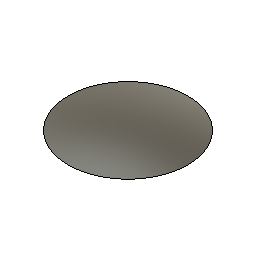
form (Autodesk Fusion 360 design; units mm, degrees)
Autodesk Fusion 360 part; units mm, degrees
sphere "Prymityw sfery1" add diameter 1500 placed x (1, 0, 0) y (0, 0, -1) z (0, 1, 0) at (0, 0, 0)
move_body "Przesuń1" bodies 1 to x (1, 0, 0) y (0, 1, 0) z (0, 0, 1) at (0, 0, -500)
move_body "Przesuń2" bodies 1 to x (1, 0, 0) y (0, 1, 0) z (0, 0, 1) at (-85, -15, -250)
sketch "Szkic3" plane through (0, 0, 0) normal (1, 0, 0) x (0, 1, 0)
  line L0 (-900, -1600) -> (967.0151, -1600)
  line L1 (967.0151, -1600) -> (967.0151, -7.311)
  line L2 (967.0151, -7.311) -> (-900, -7.311)
  line L3 (-900, -7.311) -> (-900, -1600)
  constraint horizontal L0
  constraint vertical L1
  constraint horizontal L2
  constraint vertical L3
extrude "Wyciągnięcie proste1" cut sketch "Szkic3" along normal mid plane 2000
